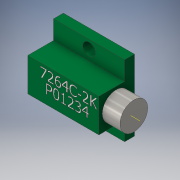
# Autodesk Inventor part: Endevco-7264C
Saved by Autodesk Inventor 2016 (Build 200138000, 138)
## iProperties
Created: 2016-06-29
Part Number: Endevco-7264C
Material: Stainless Steel
Document SubType Name: Modeling
Designer: kam42
Density: 8 g/cm^3
Appearance: Semi-Polished
Author: kam42
Autodesk Inventor part; units mm, degrees
ref_plane "YZ Plane" through (0, 0, 0) normal (1, 0, 0) x (0, 1, 0)
ref_plane "XZ Plane" through (0, 0, 0) normal (0, 1, 0) x (-1, 0, 0)
ref_plane "XY Plane" through (0, 0, 0) normal (0, 0, 1) x (1, 0, 0)
sketch "Sketch1" plane through (0, 0, 0) normal (0, 0, 1) x (1, 0, 0)
  line L0 (-5.08, -5.08) -> (5.08, -5.08)
  line L1 (5.08, -5.08) -> (5.08, 5.08)
  line L2 (5.08, 5.08) -> (-5.08, 5.08)
  line L3 (-5.08, 5.08) -> (-5.08, -5.08)
  line L4 (-5.08, -5.08) -> (5.08, 5.08) construction
  line L5 (5.08, -5.08) -> (-5.08, 5.08) construction
  circle A0 centre (0, 3.81) radius 0.9017
  line L6 (-5.08, 0) -> (5.08, 0) construction
  line L7 (0, 5.08) -> (0, -5.08) construction
  circle A1 centre (0, -3.81) radius 0.9017
  point P0 (0, 0)
  dimension "d1" = 10.16
  dimension "d2" = 10.16
  dimension "d3" = 1.8034
  dimension "d4" = 1.27
  constraints: 16 end point, 6 midpoint, 2 centre point, 2 parallel, 1 horizontal, 1 perpendicular, 1 point on line, 1 symmetric about line, 1 other
  measures "d1" distance of L1.end L2.end
  measures "d2" distance of L2.end L0.start
  measures "d3" diameter of A0
  measures "d4" distance from line of L2 A0.centre
extrude "Extrusion1" add sketch "Sketch1" along normal blind 1.397
sketch "Sketch2" plane through (0, 0, 1.397) normal (0, 0, 1) x (1, 0, 0)
  line L0 (5.08, -5.08) -> (5.08, 5.08) projected
  line L1 (-5.08, -2.3876) -> (5.08, -2.3876)
  line L2 (5.08, -2.3876) -> (5.08, 2.3876)
  line L3 (5.08, 2.3876) -> (-5.08, 2.3876)
  line L4 (-5.08, 2.3876) -> (-5.08, -2.3876)
  line L5 (-5.08, -2.3876) -> (5.08, 2.3876) construction
  line L6 (5.08, -2.3876) -> (-5.08, 2.3876) construction
  point P0 (0, 0)
  dimension "d7" = 4.7752
  constraints: 12 end point, 2 midpoint, 2 parallel, 1 horizontal, 1 perpendicular, 1 point on line
  measures "d7" distance of L3.end L1.start
extrude "Extrusion2" add sketch "Sketch2" along normal blind 3.683
sketch "Sketch3" plane through (5.08, -5.08, 0) normal (1, 0, 0) x (0, 0, -1)
  circle A0 centre (-2.6162, 5.08) radius 1.9812
  line L0 (0, 0) -> (0, 10.16) projected
  point P0 (0, 5.08)
  dimension "d10" = 3.9624
  dimension "d11" = 2.6162
  constraints: 1 centre point
  measures "d10" diameter of A0
  measures "d11" distance from line of L0 A0.centre
extrude "Extrusion3" add sketch "Sketch3" along normal blind 2.54
sketch "Sketch4" plane through (0, 0, 5.08) normal (0, 0, 1) x (1, 0, 0)
  line L0 (-3.4074, 1.996) -> (5.0034, 1.996) construction
  line L1 (5.0034, 1.996) -> (5.0034, 0.4398) construction
  line L2 (5.0034, 0.4398) -> (-3.4074, 0.4398) construction
  line L3 (-3.4074, 0.4398) -> (-3.4074, 1.996) construction
  line L4 (-2.6224, 0.309) -> (3.724, 0.309) construction
  line L5 (3.724, 0.309) -> (3.724, -1.2484) construction
  line L6 (3.724, -1.2484) -> (-2.6224, -1.2484) construction
  line L7 (-2.6224, -1.2484) -> (-2.6224, 0.309) construction
  line L8 (-2.4282, 1.7572) -> (-3.0327, 0.5696)
  line L9 (-3.0327, 0.5696) -> (-3.232, 0.5696)
  line L10 (-3.232, 0.5696) -> (-2.5935, 1.8024)
  line L11 (-2.5935, 1.8024) -> (-3.3146, 1.8024)
  line L12 (-3.3146, 1.8024) -> (-3.3146, 1.9666)
  line L13 (-3.3146, 1.9666) -> (-2.4282, 1.9666)
  line L14 (-2.4282, 1.9666) -> (-2.4282, 1.7572)
  line L15 (-1.3957, 0.5696) -> (-2.2572, 0.5696)
  line L16 (-2.2572, 0.5696) -> (-2.2572, 0.7677)
  spline S0 degree 2 poles (-2.2572, 0.7677) (-2.1644, 0.8549) (-1.9991, 1.0168) (-1.9199, 1.1039) knots 0 0 0 1 2 2 2
  spline S1 degree 2 poles (-1.9199, 1.1039) (-1.7603, 1.2794) (-1.6437, 1.49) (-1.6437, 1.6021) knots 0 0 0 1 2 2 2
  spline S2 degree 2 poles (-1.6437, 1.6021) (-1.6437, 1.6609) (-1.6799, 1.7492) (-1.7127, 1.7775) knots 0 0 0 1 2 2 2
  spline S3 degree 2 poles (-1.7127, 1.7775) (-1.7455, 1.8058) (-1.8316, 1.8341) (-1.8837, 1.8341) knots 0 0 0 1 2 2 2
  spline S4 degree 2 poles (-1.8837, 1.8341) (-1.9335, 1.8341) (-2.0354, 1.8092) (-2.0818, 1.79) knots 0 0 0 1 2 2 2
  spline S5 degree 2 poles (-2.0818, 1.79) (-2.1214, 1.7741) (-2.195, 1.7289) (-2.2176, 1.713) knots 0 0 0 1 2 2 2
  line L17 (-2.2176, 1.713) -> (-2.2278, 1.713)
  line L18 (-2.2278, 1.713) -> (-2.2278, 1.9123)
  spline S6 degree 2 poles (-2.2278, 1.9123) (-2.1701, 1.9406) (-1.9629, 1.996) (-1.8701, 1.996) knots 0 0 0 1 2 2 2
  spline S7 degree 2 poles (-1.8701, 1.996) (-1.6742, 1.996) (-1.4535, 1.7889) (-1.4535, 1.6123) knots 0 0 0 1 2 2 2
  spline S8 degree 2 poles (-1.4535, 1.6123) (-1.4535, 1.5296) (-1.492, 1.3915) (-1.5259, 1.3326) knots 0 0 0 1 2 2 2
  spline S9 degree 2 poles (-1.5259, 1.3326) (-1.5599, 1.2715) (-1.6584, 1.1515) (-1.7127, 1.0938) knots 0 0 0 1 2 2 2
  spline S10 degree 2 poles (-1.7127, 1.0938) (-1.801, 0.9975) (-2.0172, 0.7915) (-2.0818, 0.7315) knots 0 0 0 1 2 2 2
  line L19 (-2.0818, 0.7315) -> (-1.3957, 0.7315)
  line L20 (-1.3957, 0.7315) -> (-1.3957, 0.5696)
  spline S11 degree 2 poles (-0.3259, 1.0224) (-0.3259, 0.9149) (-0.3972, 0.7326) (-0.4572, 0.6715) knots 0 0 0 1 2 2 2
  spline S12 degree 2 poles (-0.4572, 0.6715) (-0.5195, 0.607) (-0.6757, 0.5402) (-0.7697, 0.5402) knots 0 0 0 1 2 2 2
  spline S13 degree 2 poles (-0.7697, 0.5402) (-0.8636, 0.5402) (-1.0187, 0.6036) (-1.0776, 0.667) knots 0 0 0 1 2 2 2
  spline S14 degree 2 poles (-1.0776, 0.667) (-1.1501, 0.7428) (-1.2316, 0.9975) (-1.2316, 1.1832) knots 0 0 0 1 2 2 2
  spline S15 degree 2 poles (-1.2316, 1.1832) (-1.2316, 1.3655) (-1.1569, 1.6587) (-1.0787, 1.7673) knots 0 0 0 1 2 2 2
  spline S16 degree 2 poles (-1.0787, 1.7673) (-1.0029, 1.8738) (-0.7629, 1.9926) (-0.6055, 1.9926) knots 0 0 0 1 2 2 2
  spline S17 degree 2 poles (-0.6055, 1.9926) (-0.5591, 1.9926) (-0.4776, 1.9836) (-0.447, 1.9734) knots 0 0 0 1 2 2 2
  line L21 (-0.447, 1.9734) -> (-0.447, 1.7934)
  line L22 (-0.447, 1.7934) -> (-0.455, 1.7934)
  spline S18 degree 2 poles (-0.455, 1.7934) (-0.481, 1.807) (-0.5761, 1.8307) (-0.6304, 1.8307) knots 0 0 0 1 2 2 2
  spline S19 degree 2 poles (-0.6304, 1.8307) (-0.8048, 1.8307) (-1.0187, 1.5953) (-1.0391, 1.3643) knots 0 0 0 1 2 2 2
  spline S20 degree 2 poles (-1.0391, 1.3643) (-0.9723, 1.4107) (-0.8319, 1.4617) (-0.7482, 1.4617) knots 0 0 0 1 2 2 2
  spline S21 degree 2 poles (-0.7482, 1.4617) (-0.6667, 1.4617) (-0.5444, 1.4289) (-0.4776, 1.379) knots 0 0 0 1 2 2 2
  spline S22 degree 2 poles (-0.4776, 1.379) (-0.4006, 1.3213) (-0.3259, 1.1424) (-0.3259, 1.0224) knots 0 0 0 1 2 2 2
  spline S23 degree 2 poles (-0.5161, 1.0145) (-0.5161, 1.1005) (-0.5614, 1.2172) (-0.6112, 1.2579) knots 0 0 0 1 2 2 2
  spline S24 degree 2 poles (-0.6112, 1.2579) (-0.6485, 1.2873) (-0.7414, 1.3066) (-0.7901, 1.3066) knots 0 0 0 1 2 2 2
  spline S25 degree 2 poles (-0.7901, 1.3066) (-0.8557, 1.3066) (-0.9791, 1.267) (-1.0391, 1.2296) knots 0 0 0 1 2 2 2
  spline S26 degree 2 poles (-1.0391, 1.2296) (-1.0402, 1.2092) (-1.0425, 1.1707) (-1.0425, 1.1413) knots 0 0 0 1 2 2 2
  spline S27 degree 2 poles (-1.0425, 1.1413) (-1.0425, 0.9964) (-0.9859, 0.8187) (-0.9429, 0.7722) knots 0 0 0 1 2 2 2
  spline S28 degree 2 poles (-0.9429, 0.7722) (-0.9033, 0.7281) (-0.8172, 0.693) (-0.7685, 0.693) knots 0 0 0 1 2 2 2
  spline S29 degree 2 poles (-0.7685, 0.693) (-0.6553, 0.693) (-0.5161, 0.8538) (-0.5161, 1.0145) knots 0 0 0 1 2 2 2
  line L23 (0.7383, 1.0496) -> (0.5718, 1.0496)
  line L24 (0.5718, 1.0496) -> (0.5718, 0.5696)
  line L25 (0.5718, 0.5696) -> (0.3918, 0.5696)
  line L26 (0.3918, 0.5696) -> (0.3918, 1.0496)
  line L27 (0.3918, 1.0496) -> (-0.2251, 1.0496)
  line L28 (-0.2251, 1.0496) -> (-0.2251, 1.2466)
  line L29 (-0.2251, 1.2466) -> (0.3998, 1.9666)
  line L30 (0.3998, 1.9666) -> (0.5718, 1.9666)
  line L31 (0.5718, 1.9666) -> (0.5718, 1.2002)
  line L32 (0.5718, 1.2002) -> (0.7383, 1.2002)
  line L33 (0.7383, 1.2002) -> (0.7383, 1.0496)
  line L34 (0.3918, 1.2002) -> (0.3918, 1.7458)
  line L35 (0.3918, 1.7458) -> (-0.078, 1.2002)
  line L36 (-0.078, 1.2002) -> (0.3918, 1.2002)
  spline S30 degree 2 poles (1.473, 0.5447) (1.3371, 0.5447) (1.1073, 0.6364) (1.0236, 0.7281) knots 0 0 0 1 2 2 2
  spline S31 degree 2 poles (1.0236, 0.7281) (0.9398, 0.8187) (0.8481, 1.0904) (0.8481, 1.267) knots 0 0 0 1 2 2 2
  spline S32 degree 2 poles (0.8481, 1.267) (0.8481, 1.4424) (0.9375, 1.7028) (1.0224, 1.799) knots 0 0 0 1 2 2 2
  spline S33 degree 2 poles (1.0224, 1.799) (1.1062, 1.893) (1.3349, 1.9915) (1.4764, 1.9915) knots 0 0 0 1 2 2 2
  spline S34 degree 2 poles (1.4764, 1.9915) (1.5466, 1.9915) (1.67, 1.9711) (1.7221, 1.9553) knots 0 0 0 1 2 2 2
  spline S35 degree 2 poles (1.7221, 1.9553) (1.7673, 1.9406) (1.8613, 1.8987) (1.9077, 1.8738) knots 0 0 0 1 2 2 2
  line L37 (1.9077, 1.8738) -> (1.9077, 1.6496)
  line L38 (1.9077, 1.6496) -> (1.893, 1.6496)
  spline S36 degree 2 poles (1.893, 1.6496) (1.8681, 1.6723) (1.7911, 1.7357) (1.7356, 1.7662) knots 0 0 0 1 2 2 2
  spline S37 degree 2 poles (1.7356, 1.7662) (1.6824, 1.7957) (1.5568, 1.833) (1.4753, 1.833) knots 0 0 0 1 2 2 2
  spline S38 degree 2 poles (1.4753, 1.833) (1.3858, 1.833) (1.2262, 1.7594) (1.1662, 1.6892) knots 0 0 0 1 2 2 2
  spline S39 degree 2 poles (1.1662, 1.6892) (1.1073, 1.6179) (1.0417, 1.4017) (1.0417, 1.267) knots 0 0 0 1 2 2 2
  spline S40 degree 2 poles (1.0417, 1.267) (1.0417, 1.1232) (1.1107, 0.916) (1.1707, 0.8447) knots 0 0 0 1 2 2 2
  spline S41 degree 2 poles (1.1707, 0.8447) (1.2296, 0.7756) (1.387, 0.7054) (1.4753, 0.7054) knots 0 0 0 1 2 2 2
  spline S42 degree 2 poles (1.4753, 0.7054) (1.5556, 0.7054) (1.6926, 0.7451) (1.7458, 0.7745) knots 0 0 0 1 2 2 2
  spline S43 degree 2 poles (1.7458, 0.7745) (1.7968, 0.8039) (1.8726, 0.8651) (1.8941, 0.8866) knots 0 0 0 1 2 2 2
  line L39 (1.8941, 0.8866) -> (1.9077, 0.8866)
  line L40 (1.9077, 0.8866) -> (1.9077, 0.6647)
  spline S44 degree 2 poles (1.9077, 0.6647) (1.8613, 0.6432) (1.7798, 0.6036) (1.7221, 0.5854) knots 0 0 0 1 2 2 2
  spline S45 degree 2 poles (1.7221, 0.5854) (1.6609, 0.5651) (1.5568, 0.5447) (1.473, 0.5447) knots 0 0 0 1 2 2 2
  line L41 (2.553, 1.096) -> (2.0243, 1.096)
  line L42 (2.0243, 1.096) -> (2.0243, 1.2658)
  line L43 (2.0243, 1.2658) -> (2.553, 1.2658)
  line L44 (2.553, 1.2658) -> (2.553, 1.096)
  line L45 (3.6002, 0.5696) -> (2.7387, 0.5696)
  line L46 (2.7387, 0.5696) -> (2.7387, 0.7677)
  spline S46 degree 2 poles (2.7387, 0.7677) (2.8315, 0.8549) (2.9968, 1.0168) (3.076, 1.1039) knots 0 0 0 1 2 2 2
  spline S47 degree 2 poles (3.076, 1.1039) (3.2357, 1.2794) (3.3523, 1.49) (3.3523, 1.6021) knots 0 0 0 1 2 2 2
  spline S48 degree 2 poles (3.3523, 1.6021) (3.3523, 1.6609) (3.316, 1.7492) (3.2832, 1.7775) knots 0 0 0 1 2 2 2
  spline S49 degree 2 poles (3.2832, 1.7775) (3.2504, 1.8058) (3.1643, 1.8341) (3.1123, 1.8341) knots 0 0 0 1 2 2 2
  spline S50 degree 2 poles (3.1123, 1.8341) (3.0624, 1.8341) (2.9606, 1.8092) (2.9141, 1.79) knots 0 0 0 1 2 2 2
  spline S51 degree 2 poles (2.9141, 1.79) (2.8745, 1.7741) (2.8009, 1.7289) (2.7783, 1.713) knots 0 0 0 1 2 2 2
  line L47 (2.7783, 1.713) -> (2.7681, 1.713)
  line L48 (2.7681, 1.713) -> (2.7681, 1.9123)
  spline S52 degree 2 poles (2.7681, 1.9123) (2.8258, 1.9406) (3.033, 1.996) (3.1258, 1.996) knots 0 0 0 1 2 2 2
  spline S53 degree 2 poles (3.1258, 1.996) (3.3217, 1.996) (3.5425, 1.7889) (3.5425, 1.6123) knots 0 0 0 1 2 2 2
  spline S54 degree 2 poles (3.5425, 1.6123) (3.5425, 1.5296) (3.504, 1.3915) (3.47, 1.3326) knots 0 0 0 1 2 2 2
  spline S55 degree 2 poles (3.47, 1.3326) (3.436, 1.2715) (3.3375, 1.1515) (3.2832, 1.0938) knots 0 0 0 1 2 2 2
  spline S56 degree 2 poles (3.2832, 1.0938) (3.1949, 0.9975) (2.9787, 0.7915) (2.9141, 0.7315) knots 0 0 0 1 2 2 2
  line L49 (2.9141, 0.7315) -> (3.6002, 0.7315)
  line L50 (3.6002, 0.7315) -> (3.6002, 0.5696)
  line L51 (4.8455, 0.5696) -> (4.6044, 0.5696)
  line L52 (4.6044, 0.5696) -> (4.0938, 1.2194)
  line L53 (4.0938, 1.2194) -> (4.0123, 1.1277)
  line L54 (4.0123, 1.1277) -> (4.0123, 0.5696)
  line L55 (4.0123, 0.5696) -> (3.8266, 0.5696)
  line L56 (3.8266, 0.5696) -> (3.8266, 1.9666)
  line L57 (3.8266, 1.9666) -> (4.0123, 1.9666)
  line L58 (4.0123, 1.9666) -> (4.0123, 1.3247)
  line L59 (4.0123, 1.3247) -> (4.5851, 1.9666)
  line L60 (4.5851, 1.9666) -> (4.8115, 1.9666)
  line L61 (4.8115, 1.9666) -> (4.233, 1.3428)
  line L62 (4.233, 1.3428) -> (4.8455, 0.5696)
  spline S57 degree 2 poles (-1.5979, -0.1416) (-1.5979, -0.2321) (-1.6624, -0.3952) (-1.7201, -0.4518) knots 0 0 0 1 2 2 2
  spline S58 degree 2 poles (-1.7201, -0.4518) (-1.7926, -0.5231) (-1.9884, -0.5967) (-2.1379, -0.5967) knots 0 0 0 1 2 2 2
  line L63 (-2.1379, -0.5967) -> (-2.2952, -0.5967)
  line L64 (-2.2952, -0.5967) -> (-2.2952, -1.1174)
  line L65 (-2.2952, -1.1174) -> (-2.4809, -1.1174)
  line L66 (-2.4809, -1.1174) -> (-2.4809, 0.2796)
  line L67 (-2.4809, 0.2796) -> (-2.1299, 0.2796)
  spline S59 degree 2 poles (-2.1299, 0.2796) (-2.0054, 0.2796) (-1.8311, 0.2388) (-1.7643, 0.1924) knots 0 0 0 1 2 2 2
  spline S60 degree 2 poles (-1.7643, 0.1924) (-1.6862, 0.1392) (-1.5979, -0.025) (-1.5979, -0.1416) knots 0 0 0 1 2 2 2
  spline S61 degree 2 poles (-1.7914, -0.1472) (-1.7914, -0.0748) (-1.8413, 0.0316) (-1.8922, 0.0656) knots 0 0 0 1 2 2 2
  spline S62 degree 2 poles (-1.8922, 0.0656) (-1.9364, 0.095) (-2.0541, 0.1188) (-2.1413, 0.1188) knots 0 0 0 1 2 2 2
  line L68 (-2.1413, 0.1188) -> (-2.2952, 0.1188)
  line L69 (-2.2952, 0.1188) -> (-2.2952, -0.4382)
  line L70 (-2.2952, -0.4382) -> (-2.1684, -0.4382)
  spline S63 degree 2 poles (-2.1684, -0.4382) (-2.0552, -0.4382) (-1.916, -0.4019) (-1.8707, -0.3544) knots 0 0 0 1 2 2 2
  spline S64 degree 2 poles (-1.8707, -0.3544) (-1.8288, -0.3125) (-1.7914, -0.214) (-1.7914, -0.1472) knots 0 0 0 1 2 2 2
  spline S65 degree 2 poles (-0.5914, -0.4189) (-0.5914, -0.7948) (-0.8099, -1.1469) (-1.0375, -1.1469) knots 0 0 0 1 2 2 2
  spline S66 degree 2 poles (-1.0375, -1.1469) (-1.2684, -1.1469) (-1.4846, -0.788) (-1.4846, -0.4201) knots 0 0 0 1 2 2 2
  spline S67 degree 2 poles (-1.4846, -0.4201) (-1.4846, -0.0419) (-1.2662, 0.3079) (-1.0375, 0.3079) knots 0 0 0 1 2 2 2
  spline S68 degree 2 poles (-1.0375, 0.3079) (-0.8077, 0.3079) (-0.5914, -0.0544) (-0.5914, -0.4189) knots 0 0 0 1 2 2 2
  spline S69 degree 2 poles (-0.8314, -0.8446) (-0.8043, -0.7755) (-0.7816, -0.5627) (-0.7816, -0.4189) knots 0 0 0 1 2 2 2
  spline S70 degree 2 poles (-0.7816, -0.4189) (-0.7816, -0.2751) (-0.8043, -0.0634) (-0.8326, 0.0079) knots 0 0 0 1 2 2 2
  spline S71 degree 2 poles (-0.8326, 0.0079) (-0.8609, 0.0792) (-0.9594, 0.1528) (-1.0375, 0.1528) knots 0 0 0 1 2 2 2
  spline S72 degree 2 poles (-1.0375, 0.1528) (-1.1156, 0.1528) (-1.2163, 0.0792) (-1.2458, 0.0056) knots 0 0 0 1 2 2 2
  spline S73 degree 2 poles (-1.2458, 0.0056) (-1.2741, -0.0657) (-1.2945, -0.2831) (-1.2945, -0.4201) knots 0 0 0 1 2 2 2
  spline S74 degree 2 poles (-1.2945, -0.4201) (-1.2945, -0.5672) (-1.2763, -0.7642) (-1.2469, -0.8412) knots 0 0 0 1 2 2 2
  spline S75 degree 2 poles (-1.2469, -0.8412) (-1.2197, -0.9136) (-1.119, -0.9918) (-1.0375, -0.9918) knots 0 0 0 1 2 2 2
  spline S76 degree 2 poles (-1.0375, -0.9918) (-0.9605, -0.9918) (-0.8597, -0.9182) (-0.8314, -0.8446) knots 0 0 0 1 2 2 2
  line L71 (0.3788, -1.1174) -> (-0.3027, -1.1174)
  line L72 (-0.3027, -1.1174) -> (-0.3027, -0.9748)
  line L73 (-0.3027, -0.9748) -> (-0.0492, -0.9748)
  line L74 (-0.0492, -0.9748) -> (-0.0492, -0.0385)
  line L75 (-0.0492, -0.0385) -> (-0.3027, -0.0385)
  line L76 (-0.3027, -0.0385) -> (-0.3027, 0.0894)
  spline S77 degree 2 poles (-0.3027, 0.0894) (-0.159, 0.0894) (-0.0231, 0.1709) (-0.0141, 0.2841) knots 0 0 0 1 2 2 2
  line L77 (-0.0141, 0.2841) -> (0.1308, 0.2841)
  line L78 (0.1308, 0.2841) -> (0.1308, -0.9748)
  line L79 (0.1308, -0.9748) -> (0.3788, -0.9748)
  line L80 (0.3788, -0.9748) -> (0.3788, -1.1174)
  line L81 (1.4973, -1.1174) -> (0.6358, -1.1174)
  line L82 (0.6358, -1.1174) -> (0.6358, -0.9193)
  spline S78 degree 2 poles (0.6358, -0.9193) (0.7286, -0.8321) (0.8939, -0.6702) (0.9731, -0.5831) knots 0 0 0 1 2 2 2
  spline S79 degree 2 poles (0.9731, -0.5831) (1.1327, -0.4076) (1.2494, -0.197) (1.2494, -0.085) knots 0 0 0 1 2 2 2
  spline S80 degree 2 poles (1.2494, -0.085) (1.2494, -0.0261) (1.2131, 0.0622) (1.1803, 0.0905) knots 0 0 0 1 2 2 2
  spline S81 degree 2 poles (1.1803, 0.0905) (1.1475, 0.1188) (1.0614, 0.1471) (1.0093, 0.1471) knots 0 0 0 1 2 2 2
  spline S82 degree 2 poles (1.0093, 0.1471) (0.9595, 0.1471) (0.8576, 0.1222) (0.8112, 0.103) knots 0 0 0 1 2 2 2
  spline S83 degree 2 poles (0.8112, 0.103) (0.7716, 0.0871) (0.698, 0.0418) (0.6754, 0.026) knots 0 0 0 1 2 2 2
  line L83 (0.6754, 0.026) -> (0.6652, 0.026)
  line L84 (0.6652, 0.026) -> (0.6652, 0.2252)
  spline S84 degree 2 poles (0.6652, 0.2252) (0.7229, 0.2535) (0.9301, 0.309) (1.0229, 0.309) knots 0 0 0 1 2 2 2
  spline S85 degree 2 poles (1.0229, 0.309) (1.2188, 0.309) (1.4395, 0.1018) (1.4395, -0.0748) knots 0 0 0 1 2 2 2
  spline S86 degree 2 poles (1.4395, -0.0748) (1.4395, -0.1574) (1.4011, -0.2955) (1.3671, -0.3544) knots 0 0 0 1 2 2 2
  spline S87 degree 2 poles (1.3671, -0.3544) (1.3331, -0.4155) (1.2346, -0.5355) (1.1803, -0.5933) knots 0 0 0 1 2 2 2
  spline S88 degree 2 poles (1.1803, -0.5933) (1.092, -0.6895) (0.8758, -0.8955) (0.8112, -0.9555) knots 0 0 0 1 2 2 2
  line L85 (0.8112, -0.9555) -> (1.4973, -0.9555)
  line L86 (1.4973, -0.9555) -> (1.4973, -1.1174)
  spline S89 degree 2 poles (2.0611, 0.1471) (2.0101, 0.1471) (1.9094, 0.1222) (1.8607, 0.103) knots 0 0 0 1 2 2 2
  spline S90 degree 2 poles (1.8607, 0.103) (1.8154, 0.0837) (1.7486, 0.043) (1.7226, 0.0249) knots 0 0 0 1 2 2 2
  line L87 (1.7226, 0.0249) -> (1.7112, 0.0249)
  line L88 (1.7112, 0.0249) -> (1.7112, 0.223)
  spline S91 degree 2 poles (1.7112, 0.223) (1.7724, 0.2558) (1.9818, 0.309) (2.0758, 0.309) knots 0 0 0 1 2 2 2
  spline S92 degree 2 poles (2.0758, 0.309) (2.1709, 0.309) (2.3124, 0.2705) (2.3701, 0.2298) knots 0 0 0 1 2 2 2
  spline S93 degree 2 poles (2.3701, 0.2298) (2.4313, 0.1856) (2.4946, 0.0577) (2.4946, -0.0284) knots 0 0 0 1 2 2 2
  spline S94 degree 2 poles (2.4946, -0.0284) (2.4946, -0.1438) (2.3429, -0.3182) (2.2365, -0.3408) knots 0 0 0 1 2 2 2
  line L89 (2.2365, -0.3408) -> (2.2365, -0.3544)
  spline S95 degree 2 poles (2.2365, -0.3544) (2.2807, -0.3635) (2.3814, -0.4042) (2.4245, -0.445) knots 0 0 0 1 2 2 2
  spline S96 degree 2 poles (2.4245, -0.445) (2.4675, -0.4846) (2.5218, -0.6114) (2.5218, -0.7031) knots 0 0 0 1 2 2 2
  spline S97 degree 2 poles (2.5218, -0.7031) (2.5218, -0.797) (2.4573, -0.9567) (2.3984, -1.0178) knots 0 0 0 1 2 2 2
  spline S98 degree 2 poles (2.3984, -1.0178) (2.3373, -1.0812) (2.1641, -1.1469) (2.0543, -1.1469) knots 0 0 0 1 2 2 2
  spline S99 degree 2 poles (2.0543, -1.1469) (1.949, -1.1469) (1.7429, -1.0959) (1.6728, -1.0608) knots 0 0 0 1 2 2 2
  line L90 (1.6728, -1.0608) -> (1.6728, -0.8627)
  line L91 (1.6728, -0.8627) -> (1.6863, -0.8627)
  spline S100 degree 2 poles (1.6863, -0.8627) (1.7452, -0.9057) (1.9445, -0.985) (2.0429, -0.985) knots 0 0 0 1 2 2 2
  spline S101 degree 2 poles (2.0429, -0.985) (2.1007, -0.985) (2.2162, -0.9487) (2.2546, -0.9069) knots 0 0 0 1 2 2 2
  spline S102 degree 2 poles (2.2546, -0.9069) (2.292, -0.865) (2.3316, -0.7653) (2.3316, -0.6895) knots 0 0 0 1 2 2 2
  spline S103 degree 2 poles (2.3316, -0.6895) (2.3316, -0.6136) (2.2875, -0.5152) (2.2479, -0.4869) knots 0 0 0 1 2 2 2
  spline S104 degree 2 poles (2.2479, -0.4869) (2.2082, -0.4585) (2.1007, -0.437) (2.0373, -0.437) knots 0 0 0 1 2 2 2
  line L92 (2.0373, -0.437) -> (1.958, -0.437)
  line L93 (1.958, -0.437) -> (1.958, -0.2819)
  line L94 (1.958, -0.2819) -> (2.0203, -0.2819)
  spline S105 degree 2 poles (2.0203, -0.2819) (2.146, -0.2819) (2.3045, -0.1619) (2.3045, -0.0476) knots 0 0 0 1 2 2 2
  spline S106 degree 2 poles (2.3045, -0.0476) (2.3045, 0.0056) (2.2637, 0.0815) (2.2309, 0.1041) knots 0 0 0 1 2 2 2
  spline S107 degree 2 poles (2.2309, 0.1041) (2.1958, 0.1279) (2.1097, 0.1471) (2.0611, 0.1471) knots 0 0 0 1 2 2 2
  line L95 (3.6313, -0.6374) -> (3.4649, -0.6374)
  line L96 (3.4649, -0.6374) -> (3.4649, -1.1174)
  line L97 (3.4649, -1.1174) -> (3.2848, -1.1174)
  line L98 (3.2848, -1.1174) -> (3.2848, -0.6374)
  line L99 (3.2848, -0.6374) -> (2.6679, -0.6374)
  line L100 (2.6679, -0.6374) -> (2.6679, -0.4404)
  line L101 (2.6679, -0.4404) -> (3.2928, 0.2796)
  line L102 (3.2928, 0.2796) -> (3.4649, 0.2796)
  line L103 (3.4649, 0.2796) -> (3.4649, -0.4869)
  line L104 (3.4649, -0.4869) -> (3.6313, -0.4869)
  line L105 (3.6313, -0.4869) -> (3.6313, -0.6374)
  line L106 (3.2848, -0.4869) -> (3.2848, 0.0588)
  line L107 (3.2848, 0.0588) -> (2.815, -0.4869)
  line L108 (2.815, -0.4869) -> (3.2848, -0.4869)
  point P0 (0, 0)
  constraints: 4 other
emboss "Emboss1" sketch "Sketch4" operation cut depth 0.0254 direction (0, 0, -1)
sketch "Sketch6" plane through (7.62, 0, 2.6162) normal (1, 0, 0) x (0, 0, -1)
  line L0 (2.6162, -5.08) -> (2.6162, 5.08) projected
  circle A0 centre (0, 0) radius 1.9812 construction
  line L1 (-1.9812, 0) -> (1.9812, 0) construction
  point P0 (2.6162, 0)
  point P1 (-0.4318, 0.254)
  dimension "d20" = 3.048
  dimension "d21" = 0.254
  constraints: 2 end point, 2 point on circle, 1 horizontal
  measures "d20" distance from line of point (-0.432, 0.254) L0
  measures "d21" distance from line of L1 point (-0.432, 0.254)
sketch "Sketch7" plane through (-5.08, -5.08, 0) normal (-1, 0, 0) x (0, 0, 1)
  point P0 (0, 5.08)
  point P1 (3.048, 5.334)
body "Solid1"
